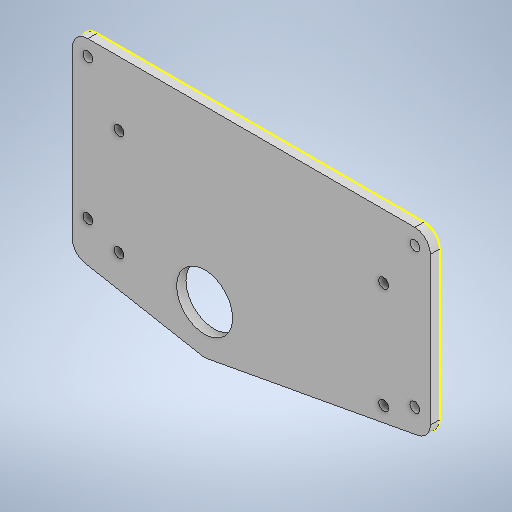
# Autodesk Inventor part: small_plate_nomotor
Saved by Autodesk Inventor 2025.1 (Build 291241000, 241)
## iProperties
Created: 2024-12-20
Part Number: small_plate_nomotor
Material: 一般
Document SubType Name: Modeling
Designer: yuki0520
Density: 1 g/cm^3
Appearance: 既定
Author: yuki0520
Autodesk Inventor part; units mm, degrees
ref_plane "YZ Plane" through (0, 0, 0) normal (1, 0, 0) x (0, 1, 0)
ref_plane "XZ Plane" through (0, 0, 0) normal (0, 1, 0) x (-1, 0, 0)
ref_plane "XY Plane" through (0, 0, 0) normal (0, 0, 1) x (1, 0, 0)
sketch "スケッチ1" plane through (0, 0, 0) normal (0, 0, 1) x (1, 0, 0)
  point P0 (0, 0)
sketch "スケッチ2" plane through (0, 0, 0) normal (0, 0, 1) x (1, 0, 0)
  line L0 (72.5, -37.5) -> (-72.5, -37.5)
  line L1 (-72.5, -37.5) -> (-72.5, 37.5)
  line L2 (-72.5, 37.5) -> (72.5, 37.5)
  line L3 (72.5, 37.5) -> (72.5, -37.5)
  line L4 (72.5, -37.5) -> (-72.5, 37.5) construction
  line L5 (-72.5, -37.5) -> (72.5, 37.5) construction
  line L6 (67.5, 32.5) -> (-67.5, 32.5)
  line L7 (-67.5, 32.5) -> (-67.5, -32.5)
  line L8 (-67.5, -32.5) -> (67.5, -32.5)
  line L9 (67.5, -32.5) -> (67.5, 32.5)
  line L10 (-67.5, 32.5) -> (-67.5, 12.5) construction
  line L11 (-69.1, 32.5) -> (-69.1, 12.5)
  line L12 (-65.9, 12.5) -> (-65.9, 32.5)
  arc A0 (-65.9, 32.5) -> (-69.1, 32.5) centre (-67.5, 32.5) ccw
  arc A1 (-69.1, 12.5) -> (-65.9, 12.5) centre (-67.5, 12.5) ccw
  line L13 (-67.5, 32.5) -> (-47.5, 32.5) construction
  line L14 (-67.5, -32.5) -> (-67.5, -12.5) construction
  line L15 (-65.9, -32.5) -> (-65.9, -12.5)
  line L16 (-69.1, -12.5) -> (-69.1, -32.5)
  arc A2 (-69.1, -32.5) -> (-65.9, -32.5) centre (-67.5, -32.5) ccw
  arc A3 (-65.9, -12.5) -> (-69.1, -12.5) centre (-67.5, -12.5) ccw
  line L17 (-67.5, -32.5) -> (-47.5, -32.5) construction
  line L18 (67.5, 32.5) -> (67.5, 12.5) construction
  line L19 (65.9, 32.5) -> (65.9, 12.5)
  line L20 (69.1, 12.5) -> (69.1, 32.5)
  arc A4 (69.1, 32.5) -> (65.9, 32.5) centre (67.5, 32.5) ccw
  arc A5 (65.9, 12.5) -> (69.1, 12.5) centre (67.5, 12.5) ccw
  line L21 (67.5, 32.5) -> (87.5, 32.5) construction
  line L22 (67.5, -32.5) -> (67.5, -12.5) construction
  line L23 (69.1, -32.5) -> (69.1, -12.5)
  line L24 (65.9, -12.5) -> (65.9, -32.5)
  arc A6 (65.9, -32.5) -> (69.1, -32.5) centre (67.5, -32.5) ccw
  arc A7 (69.1, -12.5) -> (65.9, -12.5) centre (67.5, -12.5) ccw
  line L25 (67.5, -32.5) -> (87.5, -32.5) construction
  line L26 (-72.5, -17) -> (72.5, -17)
  circle A8 centre (0, -17) radius 9
  circle A9 centre (0, -17) radius 39
  line L27 (0, 37.5) -> (0, -37.5)
  line L28 (-57.5, 37.5) -> (60, 37.5)
  line L29 (60, 37.5) -> (60, 32.5)
  line L30 (60, 32.5) -> (-60, 32.5)
  circle A10 centre (0, -155) radius 120
  circle A11 centre (-67.5, 32.5) radius 1.6
  circle A12 centre (-67.5, -12.5) radius 1.6
  circle A13 centre (67.5, 32.5) radius 1.6
  circle A14 centre (67.5, -12.5) radius 1.6
  circle A15 centre (-57.5, -17) radius 1.6
  circle A16 centre (-57.5, 17) radius 1.6
  circle A17 centre (57.5, -17) radius 1.6
  circle A18 centre (57.5, 17) radius 1.6
  line L31 (0, -32.5) -> (-72.5, -19.1)
  line L32 (0, -32.5) -> (72.5, -19.1)
  line L33 (67.5, -19.1) -> (-67.5, -19.1)
  circle A19 centre (-37.5, 32.5) radius 1.6
  circle A20 centre (-27.5, 17) radius 1.6
  circle A21 centre (-37.5, -12.5) radius 1.6
  circle A22 centre (-27.5, -17) radius 1.6
  line L34 (-42.5, 37.5) -> (-42.5, -37.5)
  point P0 (0, 0)
  point P1 (-67.5, 22.5)
  point P2 (67.5, 22.5)
  point P3 (60, 37.5)
  point P4 (-24.367, -37.5)
  point P5 (24.367, -37.5)
  point P6 (-65.9, 32.5)
  point P7 (69.1, -12.5)
  point P8 (65.9, 32.5)
  point P9 (69.1, 32.5)
  point P10 (-65.9, -12.5)
  point P11 (-35.7876, -32.5)
  point P12 (35.7876, -32.5)
  point P13 (0, 0)
  point P14 (72.5, -19.1)
  point P15 (-65.9, 32.5)
  point P16 (65.9, 32.5)
  point P17 (80, 36.6)
  point P18 (-65.9, 32.5)
  point P19 (65.9, 32.5)
  point P20 (67.5, 30.9)
  point P21 (-67.5, 30.9)
  point P22 (67.5, 10.9)
  point P23 (-67.5, 10.9)
  point P24 (-33.1776, -37.5)
  point P25 (33.1776, -37.5)
  point P26 (-42.5, 37.5)
  point P27 (-42.5, -24.6448)
  dimension "d0" = 145
  dimension "d1" = 75
  dimension "d21" = 5
  dimension "d22" = 20
  dimension "d23" = 90
  dimension "d24" = 3.2
  dimension "d25" = 20
  dimension "d26" = 90
  dimension "d27" = 3.2
  dimension "d28" = 20
  dimension "d29" = 90
  dimension "d30" = 3.2
  dimension "d31" = 20
  dimension "d32" = 90
  dimension "d33" = 3.2
  dimension "d36" = 20.5
  dimension "d37" = 18
  dimension "d38" = 78
  dimension "d42" = 120
  dimension "d43" = 60
  dimension "d45" = 240
  dimension "d46" = 138
  dimension "d47" = 3.2
  dimension "d48" = 10
  dimension "d49" = 3.2
  dimension "d50" = 10
  dimension "d51" = 17
  dimension "d52" = 17
  dimension "d54" = 5
  dimension "d57" = 30
  dimension "d62" = 30
  constraints: 78 end point, 23 centre point, 19 tangent, 16 point on circle, 13 point on line, 10 perpendicular, 9 midpoint, 9 parallel, 7 horizontal, 5 coincident, 4 collinear, 3 symmetric about line, 1 concentric, 13 other
  measures "d0" distance of L1.end L2.end
  measures "d1" distance of L0.end L1.end
  measures "d21" distance between parallel lines of L2 L6
  measures "d22" distance of L6.end L10.end
  measures "d23" angle of L10 L13
  measures "d24" diameter of A1
  measures "d25" distance of L7.end L14.end
  measures "d26" angle of L17 L14
  measures "d27" diameter of A3
  measures "d28" distance of L6.start L18.end
  measures "d29" angle of L18 L21
  measures "d30" diameter of A5
  measures "d31" distance of L8.end L22.end
  measures "d32" angle of L25 L22
  measures "d33" diameter of A7
  measures "d36" distance between parallel lines of L0 L26
  measures "d37" diameter of A8
  measures "d38" diameter of A9
  measures "d42" distance of L29.end L30.end
  measures "d43" distance from line of L27.start L29
  measures "d45" diameter of A10
  measures "d46" distance of A10.centre A9.centre
  measures "d47" diameter of A15
  measures "d48" distance from line of L7 A15.centre
  measures "d49" diameter of A16
  measures "d50" distance from line of L7 A16.centre
  measures "d51" vertical distance of point (0, 0) A16.centre
  measures "d52" distance from line of point (0, 0) L26
  measures "d54" distance edge to line of A12 L33
  measures "d57" distance of A11.centre A19.centre
  measures "d62" distance between parallel lines of L1 L34
extrude "押し出し1" add sketch "スケッチ2" along normal blind 3 contours L34 L33 A9 L31 | L31 A9 L33 A8 L27 | L27 A8 L33 A9 L32 | L34 L26 A9 L33 | A9 L33 L24 L32 | A9 L26 A22 A8 L33 | L34 L6 A19 L27 A9 A21 L26 | A8 L26 A9 L33 | A9 L26 A17 L24 L33 | L24 L33 L9 L32 | A9 A21 L27 A8 L26 A22 | L34 L2 L27 L6 A19 | A8 L27 A9 L26 | A9 L27 L6 L19 A5 L9 A7 L24 L26 A17 | L24 L26 L9 L33 | L9 L26 L23 L32 | L32 L23 L26 L3 | L2 L29 L6 L27 | L24 A14 L9 L26 | L26 L23 A7 L9 A5 L20 A4 L6 L29 L2 L3 | L26 L9 A14 L23 | A13 L9 A5 L19 | L9 A13 L20 A5
fillet "フィレット1" radius 5 5 edges at (72.5, 37.5, 1.5) (72.5, -19.1, 1.5) (0, -32.5, 1.5) (-42.5, -24.6448, 1.5) (-42.5, 37.5, 1.5)
sketch "スケッチ4" plane through (0, 0, 0) normal (0, 0, -1) x (-1, 0, 0)
  circle A0 centre (-57.5, -17) radius 1.6 projected
  circle A1 centre (-57.5, 17) radius 1.6 projected
  circle A2 centre (-67.5, 32.5) radius 1.6 projected
  circle A3 centre (-67.5, -12.5) radius 1.6 projected
  line L0 (-72.5, -14.9395) -> (-72.5, 32.5) projected
  line L1 (-67.5, 37.5) -> (37.5, 37.5) projected
  arc A4 (-67.5, 37.5) -> (-72.5, 32.5) centre (-67.5, 32.5) ccw projected
  line L2 (42.5, 32.5) -> (42.5, -20.4843) projected
  arc A5 (-0.9087, -32.332) -> (0.9087, -32.332) centre (0, -27.4153) ccw projected
  line L3 (38.4087, -25.401) -> (0.9087, -32.332) projected
  arc A6 (-72.5, -14.9395) -> (-68.4087, -19.8562) centre (-67.5, -14.9395) ccw projected
  line L4 (-0.9087, -32.332) -> (-68.4087, -19.8562) projected
  arc A7 (42.5, 32.5) -> (37.5, 37.5) centre (37.5, 32.5) ccw projected
  arc A8 (38.4087, -25.401) -> (42.5, -20.4843) centre (37.5, -20.4843) ccw projected
  point P0 (0, 0)
equation "\"d25\" = d22"
equation "\"d27\" = d24"
equation "\"d28\" = d22"
equation "\"d30\" = d24"
equation "\"d31\" = d22"
equation "\"d33\" = d24"
equation "\"d43\" = 0.5 * d42"
